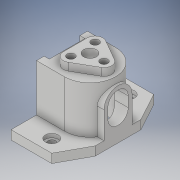
# Autodesk Inventor part: 模型1
Saved by Autodesk Inventor 2018 (Build 220112000, 112)
## iProperties
Created: 2020-05-04
Part Number: 模型1
Material: 常规
Document SubType Name: Modeling
Designer: PC
Density: 1 g/cm^3
Appearance: 默认
Author: PC
Autodesk Inventor part; units mm, degrees
ref_plane "YZ Plane" through (0, 0, 0) normal (1, 0, 0) x (0, 1, 0)
ref_plane "XZ Plane" through (0, 0, 0) normal (0, 1, 0) x (-1, 0, 0)
ref_plane "XY Plane" through (0, 0, 0) normal (0, 0, 1) x (1, 0, 0)
sketch "草图1" plane through (0, 0, 0) normal (0, 1, 0) x (-1, 0, 0)
  line L0 (22, 40) -> (22, -40)
  line L1 (0, 0) -> (22, 0) construction
  line L2 (22, 40) -> (-10, 40)
  line L3 (-10, 40) -> (-22, 18)
  line L4 (-22, 18) -> (-22, -18)
  line L5 (-22, -18) -> (-10, -40)
  line L6 (-10, -40) -> (22, -40)
  dimension "d0" = 80
  dimension "d1" = 22
  dimension "d2" = 32
  dimension "d3" = 44
  dimension "d4" = 36
  constraints: 14 end point, 2 equal length, 2 horizontal, 2 vertical, 1 midpoint, 1 perpendicular
  measures "d0" distance of L0.start L0.end
  measures "d1" distance of L1.start L1.end
  measures "d2" distance of L5.end L0.end
  measures "d3" distance between parallel lines of L4 L0
  measures "d4" distance of L3.end L4.end
extrude "拉伸1" add sketch "草图1" along normal blind 7
sketch "草图2" plane through (0, 7, 0) normal (0, 1, 0) x (1, 0, 0)
  line L0 (-44, 0) -> (0, 0) construction
  line L1 (-22, 40) -> (-22, -40) projected
  line L2 (-44, -20) -> (0, -20)
  line L3 (0, 20) -> (-44, 20)
  arc A0 (-44, 20) -> (-44, -20) centre (-44, 0) ccw
  arc A1 (0, -20) -> (0, 20) centre (0, 0) ccw
  line L4 (-22, -20) -> (-22, 20)
  point P0 (-22, 0)
  dimension "d7" = 20
  constraints: 10 end point, 4 midpoint, 4 point on circle, 4 tangent, 2 centre point, 1 horizontal, 1 parallel
  measures "d7" radius of A1
extrude "拉伸2" add sketch "草图2" along normal blind 37 contours L1 L3 A1 L2
sketch "草图3" plane through (0, 44, 0) normal (0, 1, 0) x (1, 0, 0)
  circle A0 centre (0, 0) radius 11 construction
  line L0 (0, 0) -> (-5.5, 9.5263) construction
  line L1 (0, 0) -> (-5.5, -9.5263) construction
  line L2 (0, 0) -> (11, 0) construction
  arc A1 (-2.5, 14.7224) -> (-11.5, 9.5263) centre (-5.5, 9.5263) ccw
  arc A2 (-11.5, -9.5263) -> (-2.5, -14.7224) centre (-5.5, -9.5263) ccw
  arc A3 (14, -5.1962) -> (14, 5.1962) centre (11, 0) ccw
  line L3 (-11.5, -9.5263) -> (-11.5, 9.5263)
  line L4 (14, 5.1962) -> (-2.5, 14.7224)
  line L5 (-2.5, -14.7224) -> (14, -5.1962)
  dimension "d10" = 120
  dimension "d11" = 120
  dimension "d12" = 22
  dimension "d13" = 6
  constraints: 12 end point, 9 point on circle, 5 tangent, 4 centre point, 4 coincident, 2 equal radius, 1 horizontal, 1 vertical
  measures "d10" angle of L2 L0
  measures "d11" angle of L2 L1
  measures "d12" diameter of A0
  measures "d13" radius of A2
extrude "拉伸3" add sketch "草图3" along normal blind 6
sketch "草图4" plane through (22, 0, 18) normal (1, 0, 0) x (0, 0, -1)
  line L0 (18, -28) -> (18, 28) construction
  line L1 (7, -28) -> (7, 28)
  line L2 (29, 28) -> (29, -28)
  arc A0 (7, -28) -> (29, -28) centre (18, -28) ccw
  arc A1 (29, 28) -> (7, 28) centre (18, 28) ccw
  line L3 (36, 0) -> (0, 0) projected
  line L4 (-2, 7) -> (38, 7) projected
  line L5 (7, 7) -> (29, 7)
  point P0 (18, 0)
  dimension "d16" = 28
  dimension "d17" = 11
  constraints: 10 end point, 4 point on circle, 4 point on line, 4 tangent, 2 centre point, 1 midpoint, 1 parallel, 1 vertical
  measures "d16" distance from line of L3 L0.end
  measures "d17" radius of A1
extrude "拉伸4" add sketch "草图4" against normal up to surface contours L1 A1 L2 L4
sketch "草图5" plane through (0, 7, 0) normal (0, 1, 0) x (1, 0, 0)
  line L0 (0, -30) -> (0, 30) construction
  point P0 (0, 0)
  point P1 (0, 0)
  dimension "d20" = 60
  constraints: 3 coincident, 2 end point, 1 midpoint, 1 vertical
  measures "d20" distance of L0.start L0.end
hole "孔1" at (0, 7, 30) at (0, 7, -30) direction (0, -1, 0) diameter 6 end through all counterbore diameter 10 counterbore depth 3
sketch "草图6" plane through (0, 44, 0) normal (0, 1, 0) x (1, 0, 0)
  line L0 (-26, -14) -> (-18, -14)
  line L1 (-18, -14) -> (-18, 14)
  line L2 (-18, 14) -> (-26, 14)
  line L3 (-26, 14) -> (-26, -14)
  line L4 (-22, -40) -> (-22, 40) projected
  line L5 (-26, -14) -> (-18, 14) construction
  line L6 (-18, -14) -> (-26, 14) construction
  point P0 (0, 0)
  point P1 (-22, 0)
  dimension "d28" = 28
  dimension "d29" = 4
  constraints: 12 end point, 3 midpoint, 2 parallel, 1 horizontal, 1 perpendicular
  measures "d28" distance of L2.end L0.start
  measures "d29" distance between parallel lines of L1 L4
extrude "拉伸5" cut sketch "草图6" against normal through all
sketch "草图7" plane through (0, 0, 0) normal (0, -1, 0) x (1, 0, 0)
  circle A0 centre (0, 0) radius 14
  dimension "d32" = 28
  constraints: 1 centre point, 1 coincident
  measures "d32" diameter of A0
extrude "拉伸6" cut sketch "草图7" against normal blind 40
sketch "草图8" plane through (0, 50, 0) normal (0, 1, 0) x (1, 0, 0)
  arc A0 (-2.5, 14.7224) -> (-11.5, 9.5263) centre (-5.5, 9.5263) ccw projected
  circle A1 centre (-5.5, 9.5263) radius 3
  arc A2 (-11.5, -9.5263) -> (-2.5, -14.7224) centre (-5.5, -9.5263) ccw projected
  circle A3 centre (-5.5, -9.5263) radius 3
  arc A4 (14, -5.1962) -> (14, 5.1962) centre (11, 0) ccw projected
  circle A5 centre (11, 0) radius 3
  circle A6 centre (0, 0) radius 5
  dimension "d35" = 6
  dimension "d36" = 10
  constraints: 4 centre point, 4 coincident, 2 equal radius
  measures "d35" diameter of A1
  measures "d36" diameter of A6
extrude "拉伸7" cut sketch "草图8" against normal through all
sketch "草图9" plane through (22, 0, 18) normal (1, 0, 0) x (0, 0, -1)
  line L0 (18, 0) -> (18, 24) construction
  circle A0 centre (18, 24) radius 5
  dimension "d39" = 10
  dimension "d40" = 24
  constraints: 2 end point, 1 centre point, 1 coincident, 1 vertical
  measures "d39" diameter of A0
  measures "d40" distance of L0.start L0.end
extrude "拉伸8" cut sketch "草图9" against normal through all
sketch "草图10" plane through (22, 0, 18) normal (1, 0, 0) x (0, 0, -1)
  line L0 (18, 20) -> (18, 28) construction
  circle A0 centre (18, 24) radius 5 projected
  line L1 (10, 20) -> (10, 28)
  line L2 (26, 28) -> (26, 20)
  arc A1 (10, 20) -> (26, 20) centre (18, 20) ccw
  arc A2 (26, 28) -> (10, 28) centre (18, 28) ccw
  point P0 (18, 0)
  dimension "d43" = 8
  dimension "d44" = 8
  constraints: 8 end point, 4 point on circle, 4 tangent, 2 centre point, 1 midpoint, 1 parallel, 1 vertical
  measures "d43" distance of L0.start L0.end
  measures "d44" radius of A2
extrude "拉伸9" cut sketch "草图10" against normal blind 22
